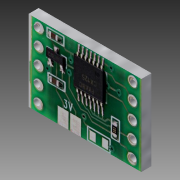
# Autodesk Inventor part: microsdadapterboard
Saved by Autodesk Inventor 2014 (Build 180170000, 170)
## iProperties
Created: 2014-06-01
Part Number: microsdadapterboard
Material: GFRC
Document SubType Name: Modeling
Designer: jose
Density: 1.7 g/cm^3
Appearance: Flat - Polished Gray
Mass: 0.59352 g
Surface Area: 5.84278 cm^2
Volume: 0.34913 cm^3
Author: jose
Autodesk Inventor part; units mm, degrees
ref_plane "YZ Plane" through (0, 0, 0) normal (1, 0, 0) x (0, 1, 0)
sketch "Sketch2" plane through (0, 0, 0) normal (0, 1, 0) x (-1, 0, 0)
  line L0 (-8.9, 6.35) -> (8.9, 6.35)
  line L1 (8.9, 6.35) -> (8.9, -6.35)
  line L2 (8.9, -6.35) -> (-8.9, -6.35)
  line L3 (-8.9, -6.35) -> (-8.9, 6.35)
  line L4 (-8.9, 6.35) -> (8.9, -6.35) construction
  line L5 (8.9, 6.35) -> (-8.9, -6.35) construction
  circle A0 centre (-7.63, 5.08) radius 0.5
  circle A1 centre (-7.63, 2.54) radius 0.5
  circle A2 centre (-7.63, -2.54) radius 0.5
  circle A3 centre (-7.63, -5.08) radius 0.5
  circle A4 centre (7.61, -5.08) radius 0.5
  circle A5 centre (7.61, -2.54) radius 0.5
  circle A6 centre (7.61, 0) radius 0.5
  circle A7 centre (7.61, 2.54) radius 0.5
  circle A8 centre (7.61, 5.08) radius 0.5
  circle A9 centre (-7.63, 0) radius 0.5
  point P0 (0, 0)
  point P1 (-7.63, -5.08)
  point P2 (-7.63, -2.54)
  point P3 (-7.63, 0)
  point P4 (-7.63, 2.54)
  point P5 (7.61, -2.54)
  point P6 (7.61, 2.54)
  dimension "d1" = 17.8
  dimension "d2" = 12.7
  dimension "d5" = 1.27
  dimension "d6" = 1.27
  dimension "d9" = 2.54
  dimension "d12" = 15.24
  dimension "d15" = 1
  dimension "d20" = 1
  dimension "d25" = 1
  dimension "d30" = 1
  dimension "d35" = 1
  dimension "d40" = 1
  dimension "d45" = 1
  dimension "d50" = 1
  dimension "d55" = 1
  dimension "d60" = 1
  constraints: 12 end point, 10 centre point, 2 horizontal, 2 midpoint, 2 parallel, 1 coincident, 1 perpendicular, 1 vertical, 9 other
  measures "d1" distance of L1.end L2.end
  measures "d2" distance of L0.end L1.end
  measures "d5" distance from line of L3 point (-7.63, -5.08)
  measures "d6" distance from line of L2 point (-7.63, -5.08)
  measures "d9" distance of point (-7.63, -5.08) point (-7.63, -2.54)
  measures "d12" distance of point (-7.63, -5.08) point (7.61, -5.08)
  measures "d15" diameter of A0
  measures "d20" diameter of A1
  measures "d25" diameter of A2
  measures "d30" diameter of A3
  measures "d35" diameter of A4
  measures "d40" diameter of A5
  measures "d45" diameter of A6
  measures "d50" diameter of A7
  measures "d55" diameter of A8
  measures "d60" diameter of A9
extrude "Extrusion2" add sketch "Sketch2" along normal mid plane 1.6
ref_plane "Work Plane1" through (0, 8.55, 0) normal (0, 1, 0) x (1, 0, 0)
sketch "Sketch3" plane through (0, 8.55, 0) normal (0, 1, 0) x (1, 0, 0)
  line L0 (-8.9372, -7.2611) -> (-8.9372, 7.6441) construction
  line L1 (-8.9372, 7.6441) -> (9.9152, 7.6441) construction
  line L2 (9.9152, 7.6441) -> (9.9152, -7.2611) construction
  line L3 (9.9152, -7.2611) -> (-8.9372, -7.2611) construction
  circle A0 centre (7.63, 0) radius 0.5 projected
  circle A1 centre (-7.61, -5.08) radius 0.5 projected
  circle A2 centre (-7.61, -2.54) radius 0.5 projected
  circle A3 centre (-7.61, 0) radius 0.5 projected
  circle A4 centre (-7.61, 2.54) radius 0.5 projected
  circle A5 centre (-7.61, 5.08) radius 0.5 projected
  circle A6 centre (7.63, 5.08) radius 0.5 projected
  circle A7 centre (7.63, 2.54) radius 0.5 projected
  circle A8 centre (7.63, -2.54) radius 0.5 projected
  circle A9 centre (7.63, -5.08) radius 0.5 projected
  line L4 (-8.9, -6.35) -> (8.9, -6.35) projected
  line L5 (8.9, -6.35) -> (8.9, 6.35) projected
  line L6 (8.9, 6.35) -> (-8.9, 6.35) projected
  line L7 (-8.9, 6.35) -> (-8.9, -6.35) projected
  point P0 (0, 0)
  constraints: 2 other
decal "Decal1"
ref_plane "Work Plane2" through (0, -20.05, 0) normal (0, -1, 0) x (1, 0, 0)
sketch "Sketch4" plane through (0, -20.05, 0) normal (0, -1, 0) x (1, 0, 0)
  line L0 (-9.0888, -7.7888) -> (-9.0888, 7.0827) construction
  line L1 (-9.0888, 7.0827) -> (9.7209, 7.0827) construction
  line L2 (9.7209, 7.0827) -> (9.7209, -7.7888) construction
  line L3 (9.7209, -7.7888) -> (-9.0888, -7.7888) construction
  circle A0 centre (7.63, 0) radius 0.5 projected
  circle A1 centre (-7.61, 5.08) radius 0.5 projected
  circle A2 centre (-7.61, 2.54) radius 0.5 projected
  circle A3 centre (-7.61, 0) radius 0.5 projected
  circle A4 centre (-7.61, -2.54) radius 0.5 projected
  circle A5 centre (-7.61, -5.08) radius 0.5 projected
  circle A6 centre (7.63, -5.08) radius 0.5 projected
  circle A7 centre (7.63, -2.54) radius 0.5 projected
  circle A8 centre (7.63, 2.54) radius 0.5 projected
  circle A9 centre (7.63, 5.08) radius 0.5 projected
  line L4 (8.9, 6.35) -> (-8.9, 6.35) projected
  line L5 (-8.9, 6.35) -> (-8.9, -6.35) projected
  line L6 (-8.9, -6.35) -> (8.9, -6.35) projected
  line L7 (8.9, -6.35) -> (8.9, 6.35) projected
  point P0 (0, 0)
  constraints: 2 other
decal "Decal2"
body "Solid2"
